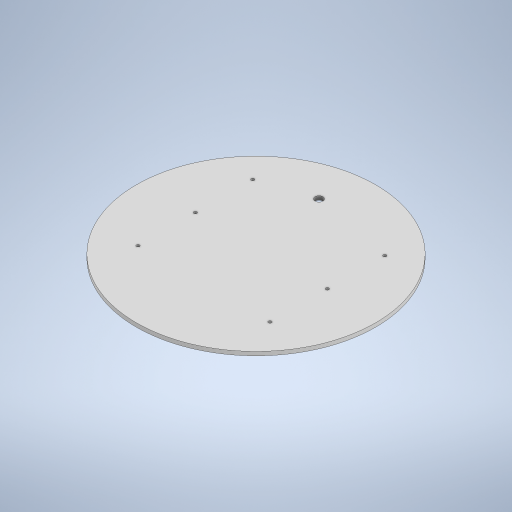
# Autodesk Inventor part: 中間台1
Saved by Autodesk Inventor 2023 (Build 270158000, 158)
## iProperties
Created: 2022-12-03
Part Number: 中間台1
Material: 一般
Document SubType Name: Modeling
Designer: RiSA
Density: 1 g/cm^3
Appearance: 既定
Author: RiSA
Autodesk Inventor part; units mm, degrees
ref_plane "YZ Plane" through (0, 0, 0) normal (1, 0, 0) x (0, 1, 0)
ref_plane "XZ Plane" through (0, 0, 0) normal (0, 1, 0) x (-1, 0, 0)
ref_plane "XY Plane" through (0, 0, 0) normal (0, 0, 1) x (1, 0, 0)
sketch "スケッチ1" plane through (0, 0, 0) normal (0, 1, 0) x (-1, 0, 0)
  circle A0 centre (0, 0) radius 125
  dimension "d0" = 250
  constraints: 1 centre point, 1 coincident
  measures "d0" diameter of A0
extrude "押し出し1" add sketch "スケッチ1" along normal blind 4
sketch "スケッチ2" plane through (0, 4, 0) normal (0, 1, 0) x (1, 0, 0)
  line L0 (75, -84.411) -> (-75, -84.411)
  line L1 (-75, -84.411) -> (-75, 95.589)
  line L2 (-75, 95.589) -> (75, 95.589)
  line L3 (75, 95.589) -> (75, -84.411)
  line L4 (75, -84.411) -> (-75, 95.589) construction
  line L5 (-75, -84.411) -> (75, 95.589) construction
  circle A0 centre (0, 0) radius 121.5
  line L6 (0, 0) -> (0, -125) construction
  circle A1 centre (0, 0) radius 125 projected
  line L7 (0, 0) -> (108.2532, 62.5) construction
  line L8 (0, 0) -> (-108.2532, 62.5) construction
  circle A2 centre (-16.75, 82.589) radius 4.1
  point P0 (0, 5.589)
  dimension "d3" = 150
  dimension "d4" = 180
  dimension "d5" = 243
  dimension "d8" = 360
  dimension "d12" = 16.75
  dimension "d13" = 13
  dimension "d14" = 8.2
  constraints: 18 end point, 2 centre point, 2 coincident, 2 midpoint, 2 parallel, 2 point on circle, 1 horizontal, 1 perpendicular, 1 vertical, 1 vertical alignment, 11 other
  measures "d3" distance of L1.end L2.end
  measures "d4" distance of L0.end L1.end
  measures "d5" diameter of A0
  measures "d12" horizontal distance of point (0, 0) point (-16.75, 82.589)
  measures "d13" distance from line of L2 point (-16.75, 82.589)
  measures "d14" diameter of A2
extrude "押し出し2" cut sketch "スケッチ2" against normal blind 4 contours A2
sketch "スケッチ4" plane through (0, 4, 0) normal (0, 1, 0) x (1, 0, 0)
  circle A0 centre (0, 0) radius 121.5
  line L0 (75, -84.411) -> (-75, -84.411)
  line L1 (-75, -84.411) -> (-75, 95.589)
  line L2 (-75, 95.589) -> (75, 95.589)
  line L3 (75, 95.589) -> (75, -84.411)
  line L4 (75, -84.411) -> (-75, 95.589) construction
  line L5 (-75, -84.411) -> (75, 95.589) construction
  line L6 (0, 0) -> (0, -29.9183)
  point P0 (0, 5.589)
  point P1 (69, -54.411)
  point P2 (69, 5.589)
  point P3 (69, 65.589)
  point P4 (-69, -54.411)
  point P5 (-69, 5.589)
  point P6 (-69, 65.589)
  dimension "d17" = 243
  dimension "d18" = 150
  dimension "d19" = 180
  dimension "d20" = 30
  dimension "d21" = 6
  dimension "d22" = 60
  dimension "d23" = 60
  constraints: 14 end point, 3 symmetric about line, 2 midpoint, 2 parallel, 2 point on circle, 1 centre point, 1 coincident, 1 horizontal, 1 perpendicular, 1 vertical
  measures "d17" diameter of A0
  measures "d18" distance of L1.end L2.end
  measures "d19" distance of L0.end L1.end
  measures "d20" distance from line of L0 point (69, -54.411)
  measures "d21" distance from line of L3 point (69, -54.411)
  measures "d22" distance of point (69, -54.411) point (69, 5.589)
  measures "d23" distance of point (69, 5.589) point (69, 65.589)
hole "穴1" at (69, 4, 54.411) at (69, 4, -5.589) at (69, 4, -65.589) at (-69, 4, -65.589) at (-69, 4, -5.589) at (-69, 4, 54.411) direction (0, -1, 0) diameter 3.2 end through all
